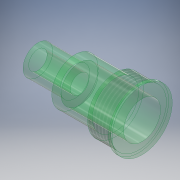
# Autodesk Inventor part: entraineur poulie 72
Saved by Autodesk Inventor 2018.1 (Build 221171000, 171)
## iProperties
Created: 2022-06-29
Part Number: entraineur poulie 72
Material: Generic
Document SubType Name: Modeling
Designer: Bureau
Density: 1 g/cm^3
Appearance: Default
Author: Bureau
Autodesk Inventor part; units mm, degrees
ref_plane "YZ Plane" through (0, 0, 0) normal (1, 0, 0) x (0, 1, 0)
ref_plane "XZ Plane" through (0, 0, 0) normal (0, 1, 0) x (-1, 0, 0)
ref_plane "XY Plane" through (0, 0, 0) normal (0, 0, 1) x (1, 0, 0)
sketch "Sketch1" plane through (0, 0, 0) normal (0, 0, 1) x (1, 0, 0)
  line L0 (0, 0) -> (10, 0)
  line L1 (0, 0) -> (0, 4)
  line L2 (0, 4) -> (18, 4)
  line L3 (18, 4) -> (18, 8)
  line L4 (18, 8) -> (45, 8)
  line L5 (45, 8) -> (45, 13)
  line L6 (45, 13) -> (43.5, 13)
  line L7 (43.5, 13) -> (43.5, 12)
  line L8 (43.5, 12) -> (33.5, 12)
  line L9 (0, 6.4082) -> (0, 4)
  line L10 (33.5, 12) -> (33.5, 10)
  line L11 (33.5, 10) -> (16, 10)
  line L12 (16, 10) -> (16, 6.4082)
  line L13 (16, 6.4082) -> (0, 6.4082)
  dimension "d0" = 10
  dimension "d18" = 4
  dimension "d19" = 18
  dimension "d20" = 4
  dimension "d21" = 27
  dimension "d22" = 5
  dimension "d23" = 1.5
  dimension "d24" = 1
  dimension "d25" = 10
  dimension "d28" = 2
  dimension "d29" = 17.5
  dimension "d30" = 16
  constraints: 28 end point, 9 perpendicular, 3 vertical, 1 horizontal
  measures "d0" distance of L0.start L0.end
  measures "d18" distance of L0.start L1.end
  measures "d19" distance of L1.end L2.end
  measures "d20" distance of L2.end L3.end
  measures "d21" distance of L3.end L4.end
  measures "d22" distance of L4.end L5.end
  measures "d23" distance of L5.end L6.end
  measures "d24" distance of L6.end L7.end
  measures "d25" distance of L7.end L8.end
  measures "d28" distance of L8.end L10.end
  measures "d29" distance of L10.end L11.end
  measures "d30" distance of L12.end L9.start
revolve "Revolution1" add sketch "Sketch1" angle 360 about axis through (0, 0, 0) along (1, 0, 0)
thread "Thread1" size "M24x1.5" class "6g" standard "ANSI Metric M Profile" full length
body "Solid1"
